tree_thing (Autodesk Fusion 360 design; units mm, degrees)
Autodesk Fusion 360 part; units mm, degrees
note: some values were not read from the file. Set by a fixed rule: which sketch regions a step uses.
sketch "Sketch1" plane through (0, 0, 0) normal (0, 1, 0) x (1, 0, 0)
  circle A0 centre (0, 0) radius 40
  circle A1 centre (0, 0) radius 47.5
  line L0 (0, 0) -> (47.5, 0)
  line L1 (0, 0) -> (-47.5, 0)
  line L2 (0, 0) -> (0, -47.5)
  line L3 (0, 0) -> (0, 47.5)
  line L4 (0, 0) -> (33.5876, 33.5876)
  dimension "d1" = 80
  dimension "d2" = 95
  dimension "d8" = 45
  constraint coincident A0.centre A1.centre
  constraint coincident A1 L0.end
  constraint horizontal L0
  constraint coincident A1 L1.end
  constraint parallel L0 L1
  constraint coincident A1 L2.end
  constraint perpendicular L0 L2
  constraint coincident A1 L3.end
  constraint parallel L2 L3
  constraint coincident A1 L4.end
  measures "d1" diameter of A0
  measures "d2" diameter of A1
  measures "d8" angle of L0 L4
extrude "Extrude1" add sketch "Sketch1" along normal blind 40 contours A0 A1 L0 L4 | A0 A1 L3 L4
ref_plane "WorkPlane1" through (40, 20, 0) normal (-0.707107, 0, 0.707107) x (0, 1, 0)
ref_plane "WorkPlane2" through (54.1421, 20, -14.1421) normal (-0.707107, 0, 0.707107) x (0, 1, 0)
sketch "Sketch2" plane through (54.1421, 20, -14.1421) normal (-0.707107, 0, 0.707107) x (0, 1, 0)
  line L0 (-20.97, 28.25) -> (19, 28.25)
  line L1 (0, 0) -> (0, 55)
  circle A0 centre (0, 28.25) radius 4
  circle A1 centre (0, 28.25) radius 7.5
  dimension "d9" = 8
  dimension "d10" = 15
  constraint horizontal L0
  constraint coincident L1.start origin
  constraint vertical L1
  constraint coincident L0 A0.centre
  constraint coincident L1 A0.centre
  constraint concentric A0 A1
  measures "d9" diameter of A0
  measures "d10" diameter of A1
extrude "Extrude2" add sketch "Sketch2" along normal blind 2 and the other way blind 10 contours L0 L1 A0 A1 | L0 L1 A0 A1 | L0 L1 A0 A1 | L0 L1 A0 A1
